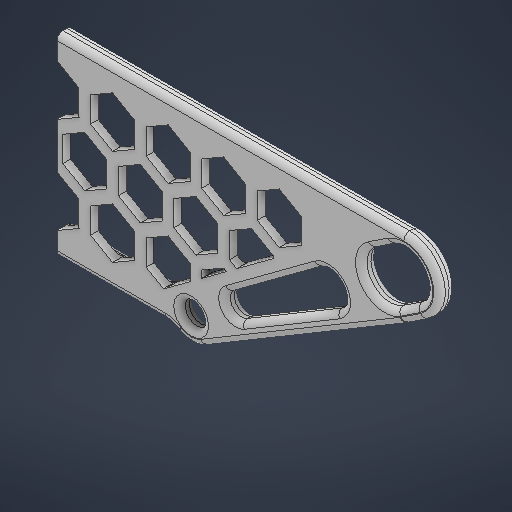
# Autodesk Inventor part: flex_battery_retainer
Saved by Autodesk Inventor 2025 (Build 290162000, 162)
## iProperties
Created: 2025-04-24
Part Number: flex_battery_retainer
Material: Všeobecné
Document SubType Name: Modeling
Designer: Simak
Density: 1 g/cm^3
Appearance: Výchozí
Author: Simak
Autodesk Inventor part; units mm, degrees
ref_plane "YZ Plane" through (0, 0, 0) normal (1, 0, 0) x (0, 1, 0)
ref_plane "XZ Plane" through (0, 0, 0) normal (0, 1, 0) x (-1, 0, 0)
ref_plane "XY Plane" through (0, 0, 0) normal (0, 0, 1) x (1, 0, 0)
sketch "Náčrt1" plane through (0, 0, 0) normal (0, 0, 1) x (1, 0, 0)
  circle A0 centre (17.302, 0) radius 1.5
  line L0 (42.2522, 16.5974) -> (44.75, 18.259) construction
  line L1 (43.9138, 14.0996) -> (46.4116, 15.7612)
  line L2 (43.0884, 20.7568) -> (40.5906, 19.0952)
  arc A1 (40.5906, 19.0952) -> (43.9138, 14.0996) centre (42.2522, 16.5974) ccw
  arc A2 (46.4116, 15.7612) -> (43.0884, 20.7568) centre (44.75, 18.259) ccw
  line L3 (47.2978, 14.429) -> (44.8, 12.7674)
  arc A3 (39.7044, 20.4274) -> (44.8, 12.7674) centre (42.2522, 16.5974) ccw
  line L4 (39.7044, 20.4274) -> (42.2022, 22.089)
  arc A4 (47.2978, 14.429) -> (42.2022, 22.089) centre (44.75, 18.259) ccw
  circle A5 centre (17.302, 0) radius 3.1
  line L5 (15.0216, -2.1) -> (0, -2.1)
  line L6 (13.3068, 0.9) -> (39.5159, 20.295)
  line L7 (18.8876, -2.6638) -> (44.6051, 12.6447)
  line L8 (22.179, 4.9774) -> (33.6716, 13.4822)
  line L9 (23.7775, 2.5744) -> (36.0629, 9.8874)
  circle A6 centre (23.0384, 3.816) radius 1.4449
  circle A7 centre (34.9574, 11.7447) radius 2.1614
  line L10 (17.302, 0) -> (23.0384, 3.816) construction
  line L11 (42.2522, 16.5974) -> (34.9574, 11.7447) construction
  line L12 (0, 0.9) -> (0, -2.1)
  line L13 (44.75, 22.859) -> (0, 22.859)
  line L14 (0, 19.859) -> (38.9266, 19.859)
  line L15 (0, 0.9) -> (13.3068, 0.9)
  line L16 (0, 22.859) -> (0, 19.859)
  point P0 (0, 0)
  point P1 (43.5011, 17.4282)
  point P2 (39.7544, 14.9358)
  point P3 (47.2478, 19.9206)
  point P4 (20.1702, 1.908)
  point P5 (21.8354, 3.0157)
  point P6 (36.757, 12.9419)
  dimension "d0" = 3
  dimension "d1" = 6
  dimension "d2" = 9
  dimension "d3" = 17.302
  dimension "d4" = 18.259
  dimension "d5" = 44.75
  dimension "d6" = 1.6
  dimension "d7" = 1.6
  dimension "d8" = 1
  dimension "d9" = 2
  dimension "d10" = 2
  dimension "d11" = 2
  dimension "d12" = 3.6
  dimension "d13" = 3
  dimension "d14" = 3
  constraints: 36 end point, 21 point on circle, 13 tangent, 8 centre point, 5 point on line, 4 horizontal, 4 parallel, 2 midpoint, 2 vertical, 1 horizontal alignment, 1 vertical alignment, 3 other
  measures "d0" diameter of A0
  measures "d1" distance between parallel lines of L2 L1
  measures "d2" distance of point (39.754, 14.936) point (47.248, 19.921)
  measures "d3" distance of point (0, 0) L10.start
  measures "d4" vertical distance of L10.start L0.end
  measures "d5" horizontal distance of point (0, 0) L0.end
  measures "d6" distance between parallel lines of L1 L3
  measures "d7" radial gap between concentric circles of A0 A5
  measures "d8" distance edge to line of A5 L5
  measures "d9" distance between parallel lines of L7 L9
  measures "d10" distance between parallel lines of L6 L8
  measures "d11" distance of point (21.835, 3.016) point (20.17, 1.908)
  measures "d12" distance of point (36.757, 12.942) point (39.754, 14.936)
  measures "d13" distance between parallel lines of L13 L14
  measures "d14" distance between parallel lines of L5 L15
extrude "Vysunutí1" add sketch "Náčrt1" along normal blind 2
fillet "Zaoblení1" radius 3 3 edges at (38.9266, 19.859, 1) (13.3068, 0.9, 1) (15.0216, -2.1, 1)
sketch "Náčrt2" plane through (0, 0, 2) normal (0, 0, 1) x (1, 0, 0)
  line L0 (0, 19.859) -> (29.8294, 19.859) projected
  line L1 (0, 19.859) -> (29.8294, 19.859) projected
  arc A0 (31.6139, 14.4475) -> (29.8294, 19.859) centre (29.8294, 16.859) ccw projected
  arc A1 (31.6139, 14.4475) -> (29.8294, 19.859) centre (29.8294, 16.859) ccw projected
  line L2 (31.6139, 14.4475) -> (14.102, 1.4885) projected
  line L3 (31.6139, 14.4475) -> (14.102, 1.4885) projected
  arc A2 (12.3175, 0.9) -> (14.102, 1.4885) centre (12.3175, 3.9) ccw projected
  arc A3 (12.3175, 0.9) -> (14.102, 1.4885) centre (12.3175, 3.9) ccw projected
  line L4 (12.3175, 0.9) -> (0, 0.9) projected
  line L5 (12.3175, 0.9) -> (0, 0.9) projected
  line L6 (0, 13.3146) -> (-2.8338, 14.9507)
  line L7 (-2.8338, 14.9507) -> (-2.8338, 18.2229)
  line L8 (-2.8338, 18.2229) -> (0, 19.859)
  line L9 (0, 19.859) -> (2.8338, 18.2229)
  line L10 (2.8338, 18.2229) -> (2.8338, 14.9507)
  line L11 (2.8338, 14.9507) -> (0, 13.3146)
  line L12 (0, 19.859) -> (29.8294, 19.859) projected
  line L13 (0, 19.859) -> (0, 0.9)
  line L14 (0, 0.9) -> (-2.8338, 2.5361)
  line L15 (-2.8338, 2.5361) -> (-2.8338, 5.8083)
  line L16 (-2.8338, 5.8083) -> (0, 7.4444)
  line L17 (0, 7.4444) -> (2.8338, 5.8083)
  line L18 (2.8338, 5.8083) -> (2.8338, 2.5361)
  line L19 (2.8338, 2.5361) -> (0, 0.9)
  line L20 (0.75, 12.0156) -> (3.5838, 13.6517)
  line L21 (3.5838, 13.6517) -> (6.4176, 12.0156)
  line L22 (6.4176, 12.0156) -> (6.4176, 8.7434)
  line L23 (6.4176, 8.7434) -> (3.5838, 7.1073)
  line L24 (3.5838, 7.1073) -> (0.75, 8.7434)
  line L25 (0.75, 8.7434) -> (0.75, 12.0156)
  line L26 (1.4169, 14.1327) -> (2.1669, 12.8336) construction
  line L27 (1.4169, 6.6263) -> (2.1669, 7.9254) construction
  line L28 (-0.75, 10.3795) -> (0.75, 10.3795) construction
  line L29 (3.5838, 1.2371) -> (6.4176, -0.399)
  line L30 (6.4176, -0.399) -> (6.4176, -3.6712)
  line L31 (6.4176, -3.6712) -> (3.5838, -5.3073)
  line L32 (3.5838, -5.3073) -> (0.75, -3.6712)
  line L33 (0.75, -3.6712) -> (0.75, -0.399)
  line L34 (0.75, -0.399) -> (3.5838, 1.2371)
  line L35 (3.5838, 19.5219) -> (0.75, 21.158)
  line L36 (0.75, 21.158) -> (0.75, 24.4302)
  line L37 (0.75, 24.4302) -> (3.5838, 26.0663)
  line L38 (3.5838, 26.0663) -> (6.4176, 24.4302)
  line L39 (6.4176, 24.4302) -> (6.4176, 21.158)
  line L40 (6.4176, 21.158) -> (3.5838, 19.5219)
  line L41 (4.3342, 14.9507) -> (4.3342, 18.2229)
  line L42 (7.168, 19.859) -> (10.0018, 18.2229)
  line L43 (4.3342, 18.2229) -> (7.168, 19.859)
  line L44 (13.5856, 24.4302) -> (13.5856, 21.158)
  line L45 (13.5856, 21.158) -> (10.7518, 19.5219)
  line L46 (10.7518, 13.6517) -> (13.5856, 12.0156)
  line L47 (10.0018, 18.2229) -> (10.0018, 14.9507)
  line L48 (10.7518, 26.0663) -> (13.5856, 24.4302)
  line L49 (8.5849, 14.1327) -> (9.3349, 12.8336) construction
  line L50 (7.918, 12.0156) -> (10.7518, 13.6517)
  line L51 (10.0018, 14.9507) -> (7.168, 13.3146)
  line L52 (10.7518, 19.5219) -> (7.918, 21.158)
  line L53 (7.918, 21.158) -> (7.918, 24.4302)
  line L54 (7.918, 24.4302) -> (10.7518, 26.0663)
  line L55 (7.168, 13.3146) -> (4.3342, 14.9507)
  line L56 (6.418, 10.3795) -> (7.918, 10.3795) construction
  line L57 (7.168, 19.859) -> (7.168, 0.9)
  line L58 (7.918, 8.7434) -> (7.918, 12.0156)
  line L59 (13.5856, 12.0156) -> (13.5856, 8.7434)
  line L60 (13.5856, 8.7434) -> (10.7518, 7.1073)
  line L61 (10.7518, 7.1073) -> (7.918, 8.7434)
  line L62 (8.5849, 6.6263) -> (9.3349, 7.9254) construction
  line L63 (4.3342, 5.8083) -> (7.168, 7.4444)
  line L64 (7.168, 7.4444) -> (10.0018, 5.8083)
  line L65 (4.3342, 2.5361) -> (4.3342, 5.8083)
  line L66 (7.168, 0.9) -> (4.3342, 2.5361)
  line L67 (10.0018, 5.8083) -> (10.0018, 2.5361)
  line L68 (10.0018, 2.5361) -> (7.168, 0.9)
  line L69 (7.918, -0.399) -> (10.7518, 1.2371)
  line L70 (10.7518, 1.2371) -> (13.5856, -0.399)
  line L71 (13.5856, -0.399) -> (13.5856, -3.6712)
  line L72 (7.918, -3.6712) -> (7.918, -0.399)
  line L73 (10.7518, -5.3073) -> (7.918, -3.6712)
  line L74 (13.5856, -3.6712) -> (10.7518, -5.3073)
  line L75 (11.5022, 14.9507) -> (11.5022, 18.2229)
  line L76 (14.336, 19.859) -> (17.1698, 18.2229)
  line L77 (11.5022, 18.2229) -> (14.336, 19.859)
  line L78 (20.7536, 24.4302) -> (20.7536, 21.158)
  line L79 (20.7536, 21.158) -> (17.9198, 19.5219)
  line L80 (17.9198, 13.6517) -> (20.7536, 12.0156)
  line L81 (17.1698, 18.2229) -> (17.1698, 14.9507)
  line L82 (17.9198, 26.0663) -> (20.7536, 24.4302)
  line L83 (15.7529, 14.1327) -> (16.5029, 12.8336) construction
  line L84 (15.086, 12.0156) -> (17.9198, 13.6517)
  line L85 (17.1698, 14.9507) -> (14.336, 13.3146)
  line L86 (17.9198, 19.5219) -> (15.086, 21.158)
  line L87 (15.086, 21.158) -> (15.086, 24.4302)
  line L88 (15.086, 24.4302) -> (17.9198, 26.0663)
  line L89 (14.336, 13.3146) -> (11.5022, 14.9507)
  line L90 (13.586, 10.3795) -> (15.086, 10.3795) construction
  line L91 (14.336, 19.859) -> (14.336, 0.9)
  line L92 (15.086, 8.7434) -> (15.086, 12.0156)
  line L93 (20.7536, 12.0156) -> (20.7536, 8.7434)
  line L94 (20.7536, 8.7434) -> (17.9198, 7.1073)
  line L95 (17.9198, 7.1073) -> (15.086, 8.7434)
  line L96 (15.7529, 6.6263) -> (16.5029, 7.9254) construction
  line L97 (11.5022, 5.8083) -> (14.336, 7.4444)
  line L98 (14.336, 7.4444) -> (17.1698, 5.8083)
  line L99 (11.5022, 2.5361) -> (11.5022, 5.8083)
  line L100 (14.336, 0.9) -> (11.5022, 2.5361)
  line L101 (17.1698, 5.8083) -> (17.1698, 2.5361)
  line L102 (17.1698, 2.5361) -> (14.336, 0.9)
  line L103 (15.086, -0.399) -> (17.9198, 1.2371)
  line L104 (17.9198, 1.2371) -> (20.7536, -0.399)
  line L105 (20.7536, -0.399) -> (20.7536, -3.6712)
  line L106 (15.086, -3.6712) -> (15.086, -0.399)
  line L107 (17.9198, -5.3073) -> (15.086, -3.6712)
  line L108 (20.7536, -3.6712) -> (17.9198, -5.3073)
  line L109 (18.6702, 14.9507) -> (18.6702, 18.2229)
  line L110 (21.504, 19.859) -> (24.3378, 18.2229)
  line L111 (18.6702, 18.2229) -> (21.504, 19.859)
  line L112 (27.9216, 24.4302) -> (27.9216, 21.158)
  line L113 (27.9216, 21.158) -> (25.0878, 19.5219)
  line L114 (25.0878, 13.6517) -> (27.9216, 12.0156)
  line L115 (24.3378, 18.2229) -> (24.3378, 14.9507)
  line L116 (25.0878, 26.0663) -> (27.9216, 24.4302)
  line L117 (22.9209, 14.1327) -> (23.6709, 12.8336) construction
  line L118 (22.254, 12.0156) -> (25.0878, 13.6517)
  line L119 (24.3378, 14.9507) -> (21.504, 13.3146)
  line L120 (25.0878, 19.5219) -> (22.254, 21.158)
  line L121 (22.254, 21.158) -> (22.254, 24.4302)
  line L122 (22.254, 24.4302) -> (25.0878, 26.0663)
  line L123 (21.504, 13.3146) -> (18.6702, 14.9507)
  line L124 (20.754, 10.3795) -> (22.254, 10.3795) construction
  line L125 (21.504, 19.859) -> (21.504, 0.9)
  line L126 (22.254, 8.7434) -> (22.254, 12.0156)
  line L127 (27.9216, 12.0156) -> (27.9216, 8.7434)
  line L128 (27.9216, 8.7434) -> (25.0878, 7.1073)
  line L129 (25.0878, 7.1073) -> (22.254, 8.7434)
  line L130 (22.9209, 6.6263) -> (23.6709, 7.9254) construction
  line L131 (18.6702, 5.8083) -> (21.504, 7.4444)
  line L132 (21.504, 7.4444) -> (24.3378, 5.8083)
  line L133 (18.6702, 2.5361) -> (18.6702, 5.8083)
  line L134 (21.504, 0.9) -> (18.6702, 2.5361)
  line L135 (24.3378, 5.8083) -> (24.3378, 2.5361)
  line L136 (24.3378, 2.5361) -> (21.504, 0.9)
  line L137 (22.254, -0.399) -> (25.0878, 1.2371)
  line L138 (25.0878, 1.2371) -> (27.9216, -0.399)
  line L139 (27.9216, -0.399) -> (27.9216, -3.6712)
  line L140 (22.254, -3.6712) -> (22.254, -0.399)
  line L141 (25.0878, -5.3073) -> (22.254, -3.6712)
  line L142 (27.9216, -3.6712) -> (25.0878, -5.3073)
  line L143 (25.8382, 14.9507) -> (25.8382, 18.2229)
  line L144 (28.672, 19.859) -> (31.5058, 18.2229)
  line L145 (25.8382, 18.2229) -> (28.672, 19.859)
  line L146 (35.0896, 24.4302) -> (35.0896, 21.158)
  line L147 (35.0896, 21.158) -> (32.2558, 19.5219)
  line L148 (32.2558, 13.6517) -> (35.0896, 12.0156)
  line L149 (31.5058, 18.2229) -> (31.5058, 14.9507)
  line L150 (32.2558, 26.0663) -> (35.0896, 24.4302)
  line L151 (30.0889, 14.1327) -> (30.8389, 12.8336) construction
  line L152 (29.422, 12.0156) -> (32.2558, 13.6517)
  line L153 (31.5058, 14.9507) -> (28.672, 13.3146)
  line L154 (32.2558, 19.5219) -> (29.422, 21.158)
  line L155 (29.422, 21.158) -> (29.422, 24.4302)
  line L156 (29.422, 24.4302) -> (32.2558, 26.0663)
  line L157 (28.672, 13.3146) -> (25.8382, 14.9507)
  line L158 (27.922, 10.3795) -> (29.422, 10.3795) construction
  line L159 (28.672, 19.859) -> (28.672, 0.9)
  line L160 (29.422, 8.7434) -> (29.422, 12.0156)
  line L161 (35.0896, 12.0156) -> (35.0896, 8.7434)
  line L162 (35.0896, 8.7434) -> (32.2558, 7.1073)
  line L163 (32.2558, 7.1073) -> (29.422, 8.7434)
  line L164 (30.0889, 6.6263) -> (30.8389, 7.9254) construction
  line L165 (25.8382, 5.8083) -> (28.672, 7.4444)
  line L166 (28.672, 7.4444) -> (31.5058, 5.8083)
  line L167 (25.8382, 2.5361) -> (25.8382, 5.8083)
  line L168 (28.672, 0.9) -> (25.8382, 2.5361)
  line L169 (31.5058, 5.8083) -> (31.5058, 2.5361)
  line L170 (31.5058, 2.5361) -> (28.672, 0.9)
  line L171 (29.422, -0.399) -> (32.2558, 1.2371)
  line L172 (32.2558, 1.2371) -> (35.0896, -0.399)
  line L173 (35.0896, -0.399) -> (35.0896, -3.6712)
  line L174 (29.422, -3.6712) -> (29.422, -0.399)
  line L175 (32.2558, -5.3073) -> (29.422, -3.6712)
  line L176 (35.0896, -3.6712) -> (32.2558, -5.3073)
  line L177 (33.0062, 14.9507) -> (33.0062, 18.2229)
  line L178 (35.84, 19.859) -> (38.6738, 18.2229)
  line L179 (33.0062, 18.2229) -> (35.84, 19.859)
  line L180 (42.2576, 24.4302) -> (42.2576, 21.158)
  line L181 (42.2576, 21.158) -> (39.4238, 19.5219)
  line L182 (39.4238, 13.6517) -> (42.2576, 12.0156)
  line L183 (38.6738, 18.2229) -> (38.6738, 14.9507)
  line L184 (39.4238, 26.0663) -> (42.2576, 24.4302)
  line L185 (37.2569, 14.1327) -> (38.0069, 12.8336) construction
  line L186 (36.59, 12.0156) -> (39.4238, 13.6517)
  line L187 (38.6738, 14.9507) -> (35.84, 13.3146)
  line L188 (39.4238, 19.5219) -> (36.59, 21.158)
  line L189 (36.59, 21.158) -> (36.59, 24.4302)
  line L190 (36.59, 24.4302) -> (39.4238, 26.0663)
  line L191 (35.84, 13.3146) -> (33.0062, 14.9507)
  line L192 (35.09, 10.3795) -> (36.59, 10.3795) construction
  line L193 (35.84, 19.859) -> (35.84, 0.9)
  line L194 (36.59, 8.7434) -> (36.59, 12.0156)
  line L195 (42.2576, 12.0156) -> (42.2576, 8.7434)
  line L196 (42.2576, 8.7434) -> (39.4238, 7.1073)
  line L197 (39.4238, 7.1073) -> (36.59, 8.7434)
  line L198 (37.2569, 6.6263) -> (38.0069, 7.9254) construction
  line L199 (33.0062, 5.8083) -> (35.84, 7.4444)
  line L200 (35.84, 7.4444) -> (38.6738, 5.8083)
  line L201 (33.0062, 2.5361) -> (33.0062, 5.8083)
  line L202 (35.84, 0.9) -> (33.0062, 2.5361)
  line L203 (38.6738, 5.8083) -> (38.6738, 2.5361)
  line L204 (38.6738, 2.5361) -> (35.84, 0.9)
  line L205 (36.59, -0.399) -> (39.4238, 1.2371)
  line L206 (39.4238, 1.2371) -> (42.2576, -0.399)
  line L207 (42.2576, -0.399) -> (42.2576, -3.6712)
  line L208 (36.59, -3.6712) -> (36.59, -0.399)
  line L209 (39.4238, -5.3073) -> (36.59, -3.6712)
  line L210 (42.2576, -3.6712) -> (39.4238, -5.3073)
  point P0 (0, 0)
  point P1 (0, 16.5868)
  point P2 (0, 4.1722)
  point P3 (3.5838, 10.3795)
  point P4 (0, 10.3795)
  point P5 (3.5838, -2.0351)
  point P6 (3.5838, 22.7941)
  point P7 (7.168, 16.5868)
  point P8 (10.7518, 22.7941)
  point P9 (7.168, 10.3795)
  point P10 (7.168, 4.1722)
  point P11 (10.7518, 10.3795)
  point P12 (10.7518, -2.0351)
  point P13 (14.336, 16.5868)
  point P14 (17.9198, 22.7941)
  point P15 (14.336, 10.3795)
  point P16 (14.336, 4.1722)
  point P17 (17.9198, 10.3795)
  point P18 (17.9198, -2.0351)
  point P19 (21.504, 16.5868)
  point P20 (25.0878, 22.7941)
  point P21 (21.504, 10.3795)
  point P22 (21.504, 4.1722)
  point P23 (25.0878, 10.3795)
  point P24 (25.0878, -2.0351)
  point P25 (28.672, 16.5868)
  point P26 (32.2558, 22.7941)
  point P27 (28.672, 10.3795)
  point P28 (28.672, 4.1722)
  point P29 (32.2558, 10.3795)
  point P30 (32.2558, -2.0351)
  point P31 (35.84, 16.5868)
  point P32 (39.4238, 22.7941)
  point P33 (35.84, 10.3795)
  point P34 (35.84, 4.1722)
  point P35 (39.4238, 10.3795)
  point P36 (39.4238, -2.0351)
  point P37 (0, 7.4444)
  point P38 (0, 0.9)
  point P39 (7.168, 0.9)
  point P40 (7.168, 0.9)
  point P41 (12.3175, 0.9)
  point P42 (13.7269, 1.2517)
  point P43 (17.1698, 3.7587)
  point P44 (18.6702, 4.869)
  point P45 (21.8671, 7.2347)
  point P46 (23.1819, 8.2077)
  point P47 (27.9216, 11.7151)
  point P48 (26.422, 10.6054)
  point P49 (29.9763, 13.2357)
  point P50 (30.9626, 13.9655)
  point P51 (31.3614, 19.4383)
  point P52 (0, 7.4444)
  point P53 (0, 0.9)
  dimension "d21" = 1.5
  dimension "d22" = 6.4176
  dimension "d23" = 1.5
  dimension "d24" = 1.5
  dimension "d27" = 7.168
  constraints: 408 end point, 17 midpoint, 7 point on line, 6 equal length, 5 vertical, 2 perpendicular, 2 vertical alignment, 1 horizontal, 445 other
  measures "d21" distance of L28.start L28.end
  measures "d22" distance between parallel lines of L13 L22
  measures "d23" distance between parallel lines of L34 L19
  measures "d24" distance between parallel lines of L9 L35
  measures "d27" distance of point (0, 16.587) point (7.168, 16.587)
extrude "Vysunutí2" add sketch "Náčrt2" against normal blind 1 contours L145 L143 L157 L159 L2 L127 L114 L118 L126 L129 L132 L125 L119 L115 L110 L0 L120 L113 | L0 A0 L2 L159 L153 L149 L144 | L113 L120 L0 | L111 L109 L123 L125 L131 L133 L2 L101 L98 L91 L85 L81 L76 L0 L86 L79 | L79 L86 L0 | L77 L75 L89 L91 L97 L99 L100 A2 L4 L70 L69 L68 L67 L64 L57 L51 L47 L42 L0 L52 L45 | L45 L52 L0 | L43 L41 L55 L57 L63 L65 L66 L4 L29 L34 L19 L18 L17 L13 L11 L10 L9 L0 L35 L40 | L40 L35 L0 | L69 L70 L4 | L4 L34 L29
fillet "Zaoblení2" radius 0.75 34 edges at (14.8143, -2.2256, 0) (17.2341, -3.0993, 0) (31.7464, 4.9904, 0) (44.7033, 12.7048, 0) (46.0489, 13.5982, 0) (49.1533, 19.5898, 0) (22.375, 22.859, 0) (6.9777, -2.1, 0) (14.8143, -2.2256, 2) (17.2341, -3.0993, 2) (31.7464, 4.9904, 2) (44.7033, 12.7048, 2) (46.0489, 13.5982, 2) (49.1533, 19.5898, 2) (22.375, 22.859, 2) (6.9777, -2.1, 2) (29.9202, 6.2309, 0) (21.8354, 3.0157, 0) (27.9253, 9.2298, 0) (36.757, 12.9419, 0) (29.9202, 6.2309, 2) (21.8354, 3.0157, 2) (27.9253, 9.2298, 2) (36.757, 12.9419, 2) (45.1627, 14.9304, 0) (39.7544, 14.9358, 0) (41.8395, 19.926, 0) (47.2478, 19.9206, 0) (45.1627, 14.9304, 2) (39.7544, 14.9358, 2) (41.8395, 19.926, 2) (47.2478, 19.9206, 2) (15.802, 0, 2) (15.802, 0, 0)
fillet "Zaoblení3" radius 0.5 17 edges at (29.2507, 19.859, 1) (29.7677, 13.0813, 1) (32.6784, 17.7985, 1) (22.858, 7.968, 0) (13.257, 1.0509, 0) (6.1587, 0.9, 0) (14.9147, 19.859, 0) (32.6784, 17.7985, 0) (22.5245, 7.7212, 1) (17.92, 4.3138, 1) (13.0438, 0.9892, 1) (9.7427, 0.9, 1) (3.584, 0.9, 1) (3.584, 19.859, 1) (10.752, 19.859, 1) (17.92, 19.859, 1) (25.088, 19.859, 1)
